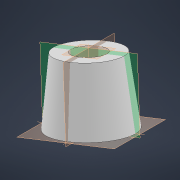
# Autodesk Inventor part: sauce bottle holder
Saved by Autodesk Inventor 2021 (Build 250183000, 183)
## iProperties
Created: 2020-10-21
Part Number: sauce bottle holder
Material: Generic
Document SubType Name: Modeling
Designer: brand
Density: 1 g/cm^3
Appearance: Default
Author: brand
## iProperties of the stored document _3DPrint.ipt
Created: 2020-10-21
Part Number: _3DPrint
Material: Generic
Document SubType Name: Modeling
Designer: brand
Density: 1 g/cm^3
Appearance: Default
Author: brand
Autodesk Inventor part; units mm, degrees
sketch "Sketch1" plane through (0, 0, 0) normal (0, 0, 1) x (1, 0, 0)
  circle A0 centre (0, 0) radius 25
  dimension "d0" = 50
  constraints: 1 centre point, 1 coincident
  measures "d0" diameter of A0
ref_plane "Work Plane2" through (0, 0, 40) normal (0, 0, 1) x (1, 0, 0)
sketch "Sketch5" plane through (0, 0, 40) normal (0, 0, 1) x (1, 0, 0)
  circle A0 centre (0, 0) radius 20
  dimension "d16" = 40
  constraints: 1 centre point, 1 coincident
  measures "d16" diameter of A0
loft "Loft2" add profiles "Sketch1", "Sketch5"
sketch "Sketch4" plane through (0, 0, 0) normal (0, 1, 0) x (-1, 0, 0)
  line L0 (-20, 40) -> (20, 40) projected
  line L1 (0, 40) -> (-10.25, 40)
  line L2 (-3.0577, 6) -> (0, 6)
  line L3 (0, 6) -> (0, 40)
  line L4 (38.1573, 12) -> (-36.662, 12) construction
  line L5 (0, -8) -> (0, 48) projected
  line L6 (-10.25, 40) -> (-10.25, 31.5)
  line L7 (-10.25, 31.5) -> (-3.0577, 6)
  point P0 (-4.75, 12)
  dimension "d22" = 10.25
  dimension "d23" = 28
  dimension "d24" = 6
  dimension "d26" = 8.5
  dimension "d27" = 4.75
  constraints: 12 end point, 3 point on line, 2 perpendicular, 1 horizontal, 1 midpoint, 1 parallel
  measures "d22" distance of L1.start L1.end
  measures "d23" distance between parallel lines of L0 L4
  measures "d24" distance between parallel lines of L4 L2
  measures "d26" distance of L1.end L6.end
  measures "d27" distance from line of L3 point (-4.75, 12)
revolve "Revolution1" cut sketch "Sketch4" angle 360 about axis through (0, 0, -10) along (0, 0, 1)
body "Solid1"
body "Solid2"
